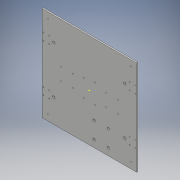
# Autodesk Inventor part: 下层板
Saved by Autodesk Inventor 2017 (Build 210142000, 142)
## iProperties
Part Number: 下层板
Material: 常规
Document SubType Name: 钣金
Designer: PANDA
Density: 1 g/cm^3
Sheet Metal Rule: 默认_mm
Appearance: 默认
Author: PANDA
Autodesk Inventor part; units mm, degrees
ref_plane "YZ Plane" through (0, 0, 0) normal (1, 0, 0) x (0, 1, 0)
ref_plane "XZ Plane" through (0, 0, 0) normal (0, 1, 0) x (-1, 0, 0)
ref_plane "XY Plane" through (0, 0, 0) normal (0, 0, 1) x (1, 0, 0)
sketch "草图1" plane through (0, 0, 0) normal (0, 1, 0) x (-1, 0, 0)
  line L0 (200, 200) -> (-200, 200)
  line L1 (-200, 200) -> (-200, -200)
  line L2 (-200, -200) -> (200, -200)
  line L3 (200, -200) -> (200, 200)
  point P0 (0, 0)
  dimension "d0" = 400
  dimension "d1" = 400
  constraints: 8 end point, 2 parallel, 1 horizontal, 1 perpendicular
  measures "d0" distance of L2.end L1.end
  measures "d1" distance of L1.end L0.end
extrude "拉伸1" add sketch "草图1" along normal blind 5
sketch "草图2" plane through (0, 5, 0) normal (0, 1, 0) x (1, 0, 0)
  circle A0 centre (175, 175) radius 1.8
  point P0 (0, 0)
  dimension "d4" = 3.6
  constraints: 1 centre point
  measures "d4" diameter of A0
extrude "拉伸2" cut sketch "草图2" against normal through all
sketch "草图3" plane through (0, 0, 0) normal (0, -1, 0) x (1, 0, 0)
  circle A0 centre (175, 175) radius 1.8
  point P0 (0, 0)
  dimension "d7" = 3.6
  constraints: 1 centre point
  measures "d7" diameter of A0
extrude "拉伸3" cut sketch "草图3" against normal through all
sketch "草图4" plane through (0, 0, 0) normal (0, -1, 0) x (1, 0, 0)
  circle A0 centre (-175, -175) radius 1.8
  point P0 (0, 0)
  dimension "d10" = 3.6
  constraints: 1 centre point
  measures "d10" diameter of A0
extrude "拉伸4" cut sketch "草图4" against normal through all
sketch "草图5" plane through (0, 0, 0) normal (0, -1, 0) x (1, 0, 0)
  circle A0 centre (-175, 175) radius 1.8
  point P0 (0, 0)
  dimension "d13" = 3.6
  constraints: 1 centre point
  measures "d13" diameter of A0
extrude "拉伸5" cut sketch "草图5" against normal through all
sketch "草图6" plane through (0, 0, 0) normal (0, -1, 0) x (1, 0, 0)
  circle A0 centre (-194, -85) radius 1.8
  point P0 (0, 0)
  dimension "d16" = 3.6
  constraints: 1 centre point
  measures "d16" diameter of A0
extrude "拉伸6" cut sketch "草图6" against normal through all
sketch "草图7" plane through (0, 0, 0) normal (0, -1, 0) x (1, 0, 0)
  circle A0 centre (-170, -85) radius 1.8
  point P0 (0, 0)
  dimension "d19" = 3.6
  constraints: 1 centre point
  measures "d19" diameter of A0
extrude "拉伸7" cut sketch "草图7" against normal through all
sketch "草图8" plane through (0, 0, 0) normal (0, -1, 0) x (1, 0, 0)
  circle A0 centre (-194, -115) radius 1.8
  point P0 (0, 0)
  dimension "d22" = 3.6
  constraints: 1 centre point
  measures "d22" diameter of A0
extrude "拉伸8" cut sketch "草图8" against normal through all
sketch "草图9" plane through (0, 0, 0) normal (0, -1, 0) x (1, 0, 0)
  circle A0 centre (-170, -115) radius 1.8
  point P0 (0, 0)
  dimension "d25" = 3.6
  constraints: 1 centre point
  measures "d25" diameter of A0
extrude "拉伸9" cut sketch "草图9" against normal through all
sketch "草图10" plane through (0, 0, 0) normal (0, -1, 0) x (1, 0, 0)
  circle A0 centre (194, 85) radius 1.8
  point P0 (0, 0)
  dimension "d28" = 3.6
  constraints: 1 centre point
  measures "d28" diameter of A0
extrude "拉伸10" cut sketch "草图10" against normal through all
sketch "草图11" plane through (0, 0, 0) normal (0, -1, 0) x (1, 0, 0)
  circle A0 centre (194, 115) radius 1.8
  point P0 (0, 0)
  dimension "d31" = 3.6
  constraints: 1 centre point
  measures "d31" diameter of A0
extrude "拉伸11" cut sketch "草图11" against normal through all
sketch "草图12" plane through (0, 0, 0) normal (0, -1, 0) x (1, 0, 0)
  circle A0 centre (170, 85) radius 1.8
  point P0 (0, 0)
  dimension "d34" = 3.6
  constraints: 1 centre point
  measures "d34" diameter of A0
extrude "拉伸12" cut sketch "草图12" against normal through all
sketch "草图13" plane through (0, 0, 0) normal (0, -1, 0) x (1, 0, 0)
  circle A0 centre (170, 115) radius 1.8
  point P0 (0, 0)
  dimension "d37" = 3.6
  constraints: 1 centre point
  measures "d37" diameter of A0
extrude "拉伸13" cut sketch "草图13" against normal through all
sketch "草图14" plane through (0, 0, 0) normal (0, -1, 0) x (1, 0, 0)
  circle A0 centre (194, -85) radius 1.8
  point P0 (0, 0)
  dimension "d40" = 3.6
  constraints: 1 centre point
  measures "d40" diameter of A0
extrude "拉伸14" cut sketch "草图14" against normal through all
sketch "草图15" plane through (0, 0, 0) normal (0, -1, 0) x (1, 0, 0)
  circle A0 centre (194, -115) radius 1.8
  point P0 (0, 0)
  dimension "d43" = 3.6
  constraints: 1 centre point
  measures "d43" diameter of A0
extrude "拉伸15" cut sketch "草图15" against normal through all
sketch "草图16" plane through (0, 0, 0) normal (0, -1, 0) x (1, 0, 0)
  circle A0 centre (170, -85) radius 1.8
  point P0 (0, 0)
  dimension "d46" = 3.6
  constraints: 1 centre point
  measures "d46" diameter of A0
extrude "拉伸16" cut sketch "草图16" against normal through all
sketch "草图17" plane through (0, 0, 0) normal (0, -1, 0) x (1, 0, 0)
  circle A0 centre (170, -115) radius 1.8
  point P0 (0, 0)
  dimension "d49" = 3.6
  constraints: 1 centre point
  measures "d49" diameter of A0
extrude "拉伸17" cut sketch "草图17" against normal through all
sketch "草图18" plane through (0, 0, 0) normal (0, -1, 0) x (1, 0, 0)
  circle A0 centre (-194, 115) radius 1.8
  point P0 (0, 0)
  dimension "d52" = 3.6
  constraints: 1 centre point
  measures "d52" diameter of A0
extrude "拉伸18" cut sketch "草图18" against normal through all
sketch "草图19" plane through (0, 0, 0) normal (0, -1, 0) x (1, 0, 0)
  circle A0 centre (-194, 85) radius 1.8
  point P0 (0, 0)
  dimension "d55" = 3.6
  constraints: 1 centre point
  measures "d55" diameter of A0
extrude "拉伸19" cut sketch "草图19" against normal through all
sketch "草图20" plane through (0, 0, 0) normal (0, -1, 0) x (1, 0, 0)
  circle A0 centre (-170, 115) radius 1.8
  point P0 (0, 0)
  dimension "d58" = 3.6
  constraints: 1 centre point
  measures "d58" diameter of A0
extrude "拉伸20" cut sketch "草图20" against normal through all
sketch "草图21" plane through (0, 0, 0) normal (0, -1, 0) x (1, 0, 0)
  circle A0 centre (-170, 85) radius 1.8
  point P0 (0, 0)
  dimension "d61" = 3.6
  constraints: 1 centre point
  measures "d61" diameter of A0
extrude "拉伸21" cut sketch "草图21" against normal through all
sketch "草图22" plane through (0, 0, 0) normal (0, -1, 0) x (1, 0, 0)
  circle A0 centre (150, 100) radius 5
  point P0 (0, 0)
  dimension "d64" = 10
  constraints: 1 centre point
  measures "d64" diameter of A0
extrude "拉伸22" cut sketch "草图22" against normal through all
sketch "草图23" plane through (0, 0, 0) normal (0, -1, 0) x (1, 0, 0)
  circle A0 centre (150, -100) radius 5
  point P0 (0, 0)
  dimension "d67" = 10
  constraints: 1 centre point
  measures "d67" diameter of A0
extrude "拉伸23" cut sketch "草图23" against normal through all
sketch "草图24" plane through (0, 0, 0) normal (0, -1, 0) x (1, 0, 0)
  circle A0 centre (-150, 100) radius 5
  point P0 (0, 0)
  dimension "d70" = 10
  constraints: 1 centre point
  measures "d70" diameter of A0
extrude "拉伸24" cut sketch "草图24" against normal through all
sketch "草图25" plane through (0, 0, 0) normal (0, -1, 0) x (1, 0, 0)
  circle A0 centre (-150, -100) radius 5
  point P0 (0, 0)
  dimension "d73" = 10
  constraints: 1 centre point
  measures "d73" diameter of A0
extrude "拉伸25" cut sketch "草图25" against normal through all
sketch "草图26" plane through (0, 0, 0) normal (0, -1, 0) x (1, 0, 0)
  circle A0 centre (24.2, 40.9) radius 1.8
  point P0 (0, 0)
  dimension "d76" = 3.6
  constraints: 1 centre point
  measures "d76" diameter of A0
extrude "拉伸26" cut sketch "草图26" against normal through all
sketch "草图27" plane through (0, 0, 0) normal (0, -1, 0) x (1, 0, 0)
  circle A0 centre (24.2, -40.9) radius 1.8
  point P0 (0, 0)
  dimension "d79" = 3.6
  constraints: 1 centre point
  measures "d79" diameter of A0
extrude "拉伸27" cut sketch "草图27" against normal through all
sketch "草图28" plane through (0, 0, 0) normal (0, -1, 0) x (1, 0, 0)
  circle A0 centre (-24.2, -40.9) radius 1.8
  point P0 (0, 0)
  dimension "d82" = 3.6
  constraints: 1 centre point
  measures "d82" diameter of A0
extrude "拉伸28" cut sketch "草图28" against normal through all
sketch "草图29" plane through (0, 0, 0) normal (0, -1, 0) x (1, 0, 0)
  circle A0 centre (-24.2, 33.9) radius 1.8
  point P0 (0, 0)
  dimension "d85" = 3.6
  constraints: 1 centre point
  measures "d85" diameter of A0
extrude "拉伸29" cut sketch "草图29" against normal through all
sketch "草图32" plane through (0, 0, 0) normal (0, -1, 0) x (1, 0, 0)
  point P0 (0, 0)
sketch "草图34" plane through (0, 0, 0) normal (0, -1, 0) x (1, 0, 0)
  point P0 (0, 0)
sketch "草图35" plane through (0, 0, 0) normal (0, -1, 0) x (1, 0, 0)
  circle A0 centre (-120.4, 26.2) radius 1.8
  point P0 (0, 0)
  dimension "d97" = 3.6
  constraints: 1 centre point
  measures "d97" diameter of A0
extrude "拉伸33" cut sketch "草图35" against normal through all
sketch "草图36" plane through (0, 0, 0) normal (0, -1, 0) x (1, 0, 0)
  circle A0 centre (-70, 26.2) radius 1.8
  point P0 (0, 0)
  dimension "d100" = 3.6
  constraints: 1 centre point
  measures "d100" diameter of A0
extrude "拉伸34" cut sketch "草图36" against normal through all
sketch "草图37" plane through (0, 0, 0) normal (0, -1, 0) x (1, 0, 0)
  circle A0 centre (70, 26.2) radius 1.8
  point P0 (0, 0)
  dimension "d103" = 3.6
  constraints: 1 centre point
  measures "d103" diameter of A0
extrude "拉伸35" cut sketch "草图37" against normal through all
sketch "草图38" plane through (0, 0, 0) normal (0, -1, 0) x (1, 0, 0)
  circle A0 centre (120.4, 26.2) radius 1.8
  point P0 (0, 0)
  dimension "d106" = 3.6
  constraints: 1 centre point
  measures "d106" diameter of A0
extrude "拉伸36" cut sketch "草图38" against normal through all
sketch "草图39" plane through (0, 0, 0) normal (0, -1, 0) x (1, 0, 0)
  circle A0 centre (-70, -26.2) radius 1.8
  point P0 (0, 0)
  dimension "d109" = 3.6
  constraints: 1 centre point
  measures "d109" diameter of A0
extrude "拉伸37" cut sketch "草图39" against normal through all
sketch "草图40" plane through (0, 0, 0) normal (0, -1, 0) x (1, 0, 0)
  circle A0 centre (70, -26.2) radius 1.8
  point P0 (0, 0)
  dimension "d112" = 3.6
  constraints: 1 centre point
  measures "d112" diameter of A0
extrude "拉伸38" cut sketch "草图40" against normal through all
sketch "草图41" plane through (0, 0, 0) normal (0, -1, 0) x (1, 0, 0)
  circle A0 centre (120.4, -26.2) radius 1.8
  point P0 (0, 0)
  dimension "d115" = 3.6
  constraints: 1 centre point
  measures "d115" diameter of A0
extrude "拉伸39" cut sketch "草图41" against normal through all
sketch "草图42" plane through (0, 0, 0) normal (0, -1, 0) x (1, 0, 0)
  circle A0 centre (-120.4, -26.2) radius 1.8
  point P0 (0, 0)
  dimension "d118" = 3.6
  constraints: 1 centre point
  measures "d118" diameter of A0
extrude "拉伸40" cut sketch "草图42" against normal through all
sketch "草图43" plane through (0, 0, 0) normal (0, -1, 0) x (1, 0, 0)
  circle A0 centre (20, -100) radius 5
  point P0 (0, 0)
  dimension "d121" = 10
  constraints: 1 centre point
  measures "d121" diameter of A0
extrude "拉伸41" cut sketch "草图43" against normal through all
sketch "草图44" plane through (0, 0, 0) normal (0, -1, 0) x (1, 0, 0)
  circle A0 centre (80, -100) radius 5
  point P0 (0, 0)
  dimension "d124" = 10
  constraints: 1 centre point
  measures "d124" diameter of A0
extrude "拉伸42" cut sketch "草图44" against normal through all
sketch "草图45" plane through (0, 0, 0) normal (0, -1, 0) x (1, 0, 0)
  circle A0 centre (20, -170) radius 5
  point P0 (0, 0)
  dimension "d127" = 10
  constraints: 1 centre point
  measures "d127" diameter of A0
extrude "拉伸43" cut sketch "草图45" against normal through all
sketch "草图46" plane through (0, 0, 0) normal (0, -1, 0) x (1, 0, 0)
  circle A0 centre (80, -170) radius 5
  point P0 (0, 0)
  dimension "d130" = 10
  constraints: 1 centre point
  measures "d130" diameter of A0
extrude "拉伸44" cut sketch "草图46" against normal through all
sketch "草图47" plane through (0, 0, 0) normal (0, -1, 0) x (1, 0, 0)
  point P0 (0, 0)
equation "\"折弯半径\" = 厚度"
equation "\"折弯释压宽度\" = 厚度"
equation "\"折弯释压深度\" = 0.5 * 厚度"
equation "\"拐角释压尺寸\" = 4 * 厚度"
equation "\"最小余量\" = 2 * 厚度"
equation "\"过渡半径\" = 折弯半径"
equation "\"Jacobi半径尺寸\" = 折弯半径"
equation "\"间隙大小\" = 厚度"
equation "\"厚度\" = 0.5"
